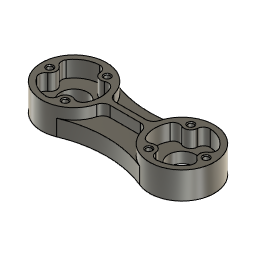
A03-03_Chen_CAM_3.f3d (Autodesk Fusion 360 design; units mm, degrees)
Autodesk Fusion 360 part; units mm, degrees
sketch "Sketch1" plane through (0, 0, 0) normal (0, 0, 1) x (1, 0, 0)
  circle A0 centre (-31.75, 0) radius 19.05
  arc A1 (0, -12.7) -> (-24.4231, -17.5846) centre (0, -76.2) ccw
  arc A2 (-24.4231, 17.5846) -> (0, 12.7) centre (0, 76.2) ccw
  line L0 (0, 12.7) -> (0, -12.7)
  dimension "d1" = 38.1
  dimension "d6" = 127
  dimension "d39" = 31.75
  constraint tangent A0 A1
  constraint equal A1 A2
  constraint coincident A0 A1.end
  constraint coincident A0 A2.start
  constraint horizontal origin A0.centre
  constraint tangent A0 A2
  constraint vertical A2.centre A1.centre
  constraint midpoint origin L0
  constraint vertical L0
  constraint coincident A2.centre L0
  measures "d1" diameter of A0
  measures "d6" diameter of A2
  measures "d39" distance of A0.centre L0
extrude "Extrude1" add sketch "Sketch1" along normal mid plane 15.875 makes body 1
sketch "Sketch2" plane through (0, 0, 7.9375) normal (0, 0, 1) x (-1, 0, 0)
  arc A0 (24.4231, -17.5846) -> (24.4231, 17.5846) centre (31.75, 0) ccw
  arc A1 (0, 12.7) -> (24.4231, 17.5846) centre (0, 76.2) ccw
  arc A2 (24.4231, -17.5846) -> (0, -12.7) centre (0, -76.2) ccw
  circle A3 centre (31.75, 0) radius 15.875
  line L0 (0, 12.7) -> (0, -12.7)
  dimension "d7" = 31.75
  constraint concentric A0 A3
  measures "d7" diameter of A3
extrude "Extrude2" cut sketch "Sketch2" against normal blind 9.525 contours A3 bodies 1
sketch "Sketch3" plane through (0, 0, 7.9375) normal (0, 0, 1) x (-1, 0, 0)
  circle A0 centre (31.75, 0) radius 15.875
  arc A1 (24.4231, -17.5846) -> (24.4231, 17.5846) centre (31.75, 0) ccw
  arc A2 (0, 12.7) -> (24.4231, 17.5846) centre (0, 76.2) ccw
  arc A3 (24.4231, -17.5846) -> (0, -12.7) centre (0, -76.2) ccw
  circle A4 centre (31.75, 0) radius 19.05
  arc A5 (24.4231, -17.5846) -> (24.4231, 17.5846) centre (31.75, 0) ccw
  line L0 (31.75, 0) -> (0, 0)
  line L1 (0, 12.7) -> (0, -12.7)
  line L2 (31.75, -1.5875) -> (0, -1.5875)
  line L3 (31.75, 1.5875) -> (0, 1.5875)
  dimension "d10" = 1.5875
  dimension "d40" = 3.175
  constraint concentric A0 A4
  constraint equal A4 A5
  constraint coincident A0.centre A1.centre
  constraint parallel L0 L2
  constraint coincident L1 L2.end
  measures "d40" distance of L2 L3
extrude "Extrude3" cut sketch "Sketch3" against normal blind 6.35 contours A2 A4 L1 L3 | A3 A4 L1 L2 bodies 1
fillet "Fillet1" radius 4.6228 2 edges at (-12.7663, 1.5875, 4.7625) (-12.7663, -1.5875, 4.7625) on bodies 1
sketch "Sketch4" plane through (0, 0, -1.5875) normal (0, 0, 1) x (-1, 0, 0)
  circle A0 centre (-31.75, 0) radius 7.9375
  circle A1 centre (31.75, 0) radius 7.9375
  circle A2 centre (31.75, 0) radius 15.875
  circle A3 centre (31.75, 0) radius 15.875
  dimension "d16" = 15.875
  constraint equal A0 A1
  constraint concentric A1 A2
  measures "d16" diameter of A0
extrude "Extrude4" cut sketch "Sketch4" against normal blind 13.5382 contours A0 | A1 bodies 1
sketch "Sketch5" plane through (0, 0, 7.9375) normal (0, 0, 1) x (-1, 0, 0)
  line L0 (0, -1.5875) -> (8.9063, -1.5875)
  arc A0 (13.3672, -4.9976) -> (8.9063, -1.5875) centre (8.9063, -6.2103) ccw
  arc A1 (8.9063, 1.5875) -> (13.3672, 4.9976) centre (8.9063, 6.2103) ccw
  line L1 (8.9063, 1.5875) -> (0, 1.5875)
  circle A2 centre (31.75, 0) radius 15.875
  circle A3 centre (46.0375, 0) radius 3.9688
  circle A4 centre (31.75, 0) radius 7.9375
  circle A5 centre (24.6063, 12.3733) radius 3.9688
  circle A6 centre (24.6062, -12.3733) radius 3.9688
  line L2 (0, 1.5875) -> (0, -1.5875)
  arc A7 (13.3672, -4.9976) -> (13.3672, 4.9976) centre (31.75, 0) ccw
  dimension "d19" = 7.9375
  dimension "d26" = 14.2875
  dimension "d32" = 360
  constraint horizontal origin A3.centre
  measures "d19" diameter of A3
  measures "d26" distance of A2.centre A3.centre
extrude "Extrude6" add sketch "Sketch5" against normal through all of body 1 contours A2 A3 | A2 A5 | A2 A6 picked at (45.9307, -1.0842) picked at (23.3161, 11.6335) picked at (23.3161, -11.6335) bodies 1
fillet "Fillet3" radius 3.81 6 edges at (-20.7478, -11.4441, 3.175) (-27.3402, -15.2502, 3.175) (-27.3402, 15.2502, 3.175) (-20.7478, 11.4441, 3.175) (-47.162, -3.8061, 3.175) (-47.162, 3.8061, 3.175) on bodies 1
sketch "Sketch6" plane through (0, 0, 7.9375) normal (0, 0, 1) x (-1, 0, 0)
  arc A0 (17.6072, 7.2109) -> (17.6072, -7.2109) centre (31.75, 0) ccw
  arc A1 (22.7671, 8.8565) -> (17.6072, 7.2109) centre (21.0015, 5.4803) ccw
  arc A2 (22.7671, 8.8565) -> (28.5715, 12.2077) centre (24.6063, 12.3733) ccw
  arc A3 (32.5766, 15.8535) -> (28.5715, 12.2077) centre (32.3782, 12.0486) ccw
  arc A4 (45.0662, 8.6426) -> (32.5766, 15.8535) centre (31.75, 0) ccw
  arc A5 (43.9114, 3.3512) -> (45.0662, 8.6426) centre (41.8703, 6.5684) ccw
  arc A6 (43.9114, 3.3512) -> (43.9114, -3.3512) centre (46.0375, 0) ccw
  arc A7 (45.0662, -8.6426) -> (43.9114, -3.3512) centre (41.8703, -6.5684) ccw
  arc A8 (32.5766, -15.8535) -> (45.0662, -8.6426) centre (31.75, 0) ccw
  arc A9 (28.5715, -12.2077) -> (32.5766, -15.8535) centre (32.3782, -12.0486) ccw
  arc A10 (28.5715, -12.2077) -> (22.7671, -8.8565) centre (24.6062, -12.3733) ccw
  arc A11 (17.6072, -7.2109) -> (22.7671, -8.8565) centre (21.0015, -5.4803) ccw
  circle A12 centre (24.6062, -12.3733) radius 1.5875
  circle A13 centre (46.0375, 0) radius 1.5875
  circle A14 centre (24.6063, 12.3733) radius 1.5875
  arc A15 (13.3672, -4.9976) -> (13.3672, 4.9976) centre (31.75, 0) ccw
  arc A16 (8.9063, 1.5875) -> (13.3672, 4.9976) centre (8.9063, 6.2103) ccw
  line L0 (8.9063, 1.5875) -> (0, 1.5875)
  line L1 (0, 1.5875) -> (0, -1.5875)
  line L2 (0, -1.5875) -> (8.9063, -1.5875)
  arc A17 (13.3672, -4.9976) -> (8.9063, -1.5875) centre (8.9063, -6.2103) ccw
  dimension "d35" = 3.175
  constraint concentric A10 A12
  constraint coincident A6.centre A13.centre
  constraint concentric A2 A14
  constraint equal A13 A14
  constraint equal A12 A14
  measures "d35" diameter of A12
extrude "Extrude7" cut sketch "Sketch6" against normal through all contours A12 | A13 | A14 bodies 1
chamfer "Chamfer1" distance 0.508 angle 45 6 edges at (-23.1262, 11.7993, 7.9375) (-44.5574, -0.5741, 7.9375) (-23.1262, -12.9474, 7.9375) (-23.1262, -11.7993, -7.9375) (-44.5574, 0.5741, -7.9375) (-23.1262, 12.9474, -7.9375) on bodies 1
mirror "Mirror3" about plane through (0, 12.7, 0) normal (1, 0, 0) of bodies 1 makes body 2
combine "Combine1" operation add target body 1 tool bodies 2
sketch "Sketch8" plane through (0, 0, -7.9375) normal (0, 0, -1) x (1, 0, 0)
  circle A0 centre (24.6063, 12.3733) radius 2.0955
  circle A1 centre (46.0375, 0) radius 2.0955
  circle A2 centre (-46.0375, 0) radius 2.0955
  circle A3 centre (-24.6063, 12.3733) radius 2.0955
  circle A4 centre (-24.6062, -12.3733) radius 2.0955
  arc A5 (-24.4231, 17.5846) -> (-24.4231, -17.5846) centre (-31.75, 0) ccw
  arc A6 (24.4231, -17.5846) -> (-24.4231, -17.5846) centre (0, -76.2) ccw
  arc A7 (-24.4231, 17.5846) -> (24.4231, 17.5846) centre (0, 76.2) ccw
  arc A8 (24.4231, -17.5846) -> (24.4231, 17.5846) centre (31.75, 0) ccw
  circle A9 centre (-31.75, 0) radius 19.05
  circle A10 centre (31.75, 0) radius 19.05
  arc A11 (25.6442, -14.6538) -> (25.6442, 14.6538) centre (31.75, 0) ccw
  arc A12 (-25.6442, 14.6538) -> (25.6442, 14.6538) centre (0, 76.2) ccw
  arc A13 (-25.6442, 14.6538) -> (-25.6442, -14.6538) centre (-31.75, 0) ccw
  arc A14 (25.6442, -14.6538) -> (-25.6442, -14.6538) centre (0, -76.2) ccw
  circle A15 centre (24.6062, -12.3733) radius 2.0955
  circle A16 centre (31.75, 0) radius 7.9375
  arc A17 (-24.4231, 17.5846) -> (-24.4231, -17.5846) centre (-31.75, 0) ccw
  arc A18 (24.4231, -17.5846) -> (-24.4231, -17.5846) centre (0, -76.2) ccw
  arc A19 (24.4231, -17.5846) -> (24.4231, 17.5846) centre (31.75, 0) ccw
  arc A20 (-24.4231, 17.5846) -> (24.4231, 17.5846) centre (0, 76.2) ccw
  circle A21 centre (-31.75, 0) radius 7.9375
  constraint tangent A13 A14
  constraint tangent A12 A13
  constraint tangent A11 A12
  constraint tangent A11 A14
extrude "Extrude8" cut sketch "Sketch8" against normal blind 6.35 contours A9 A10 A12 A14 bodies 1
fillet "Fillet4" radius 3.81 4 edges at (-16.6722, -11.6431, -4.7625) (-16.6722, 11.6431, -4.7625) (16.6722, 11.6431, -4.7625) (16.6722, -11.6431, -4.7625) on bodies 1
sketch "Sketch9" plane through (0, 0, 7.9375) normal (0, 0, 1) x (-1, 0, 0)
  arc A0 (-22.7671, -8.8565) -> (-17.6072, -7.2109) centre (-21.0015, -5.4803) ccw construction
  arc A1 (-22.7671, -8.8565) -> (-28.5715, -12.2077) centre (-24.6062, -12.3733) ccw construction
  arc A2 (-32.5766, -15.8535) -> (-28.5715, -12.2077) centre (-32.3782, -12.0486) ccw construction
  arc A3 (-43.9114, -3.3512) -> (-45.0662, -8.6426) centre (-41.8703, -6.5684) ccw construction
  arc A4 (-43.9114, -3.3512) -> (-43.9114, 3.3512) centre (-46.0375, 0) ccw construction
  arc A5 (-45.0662, 8.6426) -> (-43.9114, 3.3512) centre (-41.8703, 6.5684) ccw construction
  arc A6 (-32.5766, 15.8535) -> (-45.0662, 8.6426) centre (-31.75, 0) ccw construction
  arc A7 (-28.5715, 12.2077) -> (-32.5766, 15.8535) centre (-32.3782, 12.0486) ccw construction
  arc A8 (-28.5715, 12.2077) -> (-22.7671, 8.8565) centre (-24.6063, 12.3733) ccw construction
  arc A9 (-17.6072, 7.2109) -> (-22.7671, 8.8565) centre (-21.0015, 5.4803) ccw construction
  arc A10 (22.7671, 8.8565) -> (17.6072, 7.2109) centre (21.0015, 5.4803) ccw construction
  arc A11 (22.7671, 8.8565) -> (28.5715, 12.2077) centre (24.6063, 12.3733) ccw construction
  arc A12 (32.5766, 15.8535) -> (28.5715, 12.2077) centre (32.3782, 12.0486) ccw construction
  arc A13 (45.0662, 8.6426) -> (32.5766, 15.8535) centre (31.75, 0) ccw construction
  arc A14 (43.9114, 3.3512) -> (45.0662, 8.6426) centre (41.8703, 6.5684) ccw construction
  arc A15 (43.9114, 3.3512) -> (43.9114, -3.3512) centre (46.0375, 0) ccw construction
  arc A16 (45.0662, -8.6426) -> (43.9114, -3.3512) centre (41.8703, -6.5684) ccw construction
  arc A17 (32.5766, -15.8535) -> (45.0662, -8.6426) centre (31.75, 0) ccw construction
  arc A18 (28.5715, -12.2077) -> (32.5766, -15.8535) centre (32.3782, -12.0486) ccw construction
  arc A19 (28.5715, -12.2077) -> (22.7671, -8.8565) centre (24.6062, -12.3733) ccw construction
  arc A20 (17.6072, -7.2109) -> (22.7671, -8.8565) centre (21.0015, -5.4803) ccw construction
  line L0 (50.8, -19.05) -> (-50.8, -19.05) construction
  line L1 (-50.8, -19.05) -> (-50.8, 19.05) construction
  line L2 (-50.8, 19.05) -> (50.8, 19.05) construction
  line L3 (50.8, 19.05) -> (50.8, -19.05) construction
  circle A21 centre (24.6063, 12.3733) radius 2.0955
  line L4 (-53.975, 22.225) -> (53.975, 22.225)
  line L5 (53.975, 22.225) -> (53.975, -22.225)
  line L6 (53.975, -22.225) -> (-53.975, -22.225)
  line L7 (-53.975, -22.225) -> (-53.975, 22.225)
  circle A22 centre (-24.6063, 12.3733) radius 2.0955
  circle A23 centre (-24.6062, -12.3733) radius 2.0955
  arc A24 (-17.6072, -7.2109) -> (-17.6072, 7.2109) centre (-31.75, 0) ccw
  arc A25 (-45.0662, -8.6426) -> (-32.5766, -15.8535) centre (-31.75, 0) ccw
  circle A26 centre (-46.0375, 0) radius 2.0955
  circle A27 centre (46.0375, 0) radius 2.0955
  arc A28 (13.3672, -4.9976) -> (13.3672, 4.9976) centre (31.75, 0) ccw
  arc A29 (8.9063, 1.5875) -> (13.3672, 4.9976) centre (8.9063, 6.2103) ccw
  line L8 (8.9063, 1.5875) -> (-8.9063, 1.5875)
  arc A30 (-13.3672, 4.9976) -> (-8.9063, 1.5875) centre (-8.9063, 6.2103) ccw
  arc A31 (-13.3672, 4.9976) -> (-13.3672, -4.9976) centre (-31.75, 0) ccw
  arc A32 (-8.9063, -1.5875) -> (-13.3672, -4.9976) centre (-8.9063, -6.2103) ccw
  line L9 (-8.9063, -1.5875) -> (8.9063, -1.5875)
  arc A33 (13.3672, -4.9976) -> (8.9063, -1.5875) centre (8.9063, -6.2103) ccw
  arc A34 (17.6072, 7.2109) -> (17.6072, -7.2109) centre (31.75, 0) ccw
  circle A35 centre (24.6062, -12.3733) radius 2.0955
  dimension "d48" = 3.175
  constraint horizontal L0
  constraint vertical L1
  constraint horizontal L2
  constraint vertical L3
equation "d4 = 0.625 in / 2"
